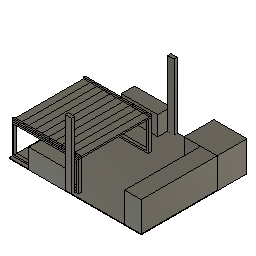
jumpy_camper_build (Autodesk Fusion 360 design; units mm, degrees)
part number: 2026-07-06-21-50-36-791
Autodesk Fusion 360 part; units mm, degrees
note: some values were not read from the file. Set by a fixed rule: which sketch regions a step uses.
sketch "Sketch1" plane through (0, 0, 0) normal (0, 0, 1) x (1, 0, 0)
  line L0 (0, 0) -> (2000, 0)
  line L1 (2000, 0) -> (2000, 1600)
  line L2 (2000, 1600) -> (0, 1600)
  line L3 (0, 1600) -> (0, 0)
  line L4 (2000, 800) -> (0, 800) construction
  line L5 (298.7393, 1600) -> (850, 1600)
  line L6 (850, 1600) -> (850, 1400)
  line L7 (850, 1400) -> (298.7393, 1400)
  line L8 (298.7393, 1400) -> (298.7393, 1600)
  line L9 (298.7393, 0) -> (850, 0)
  line L10 (850, 0) -> (850, 200)
  line L11 (850, 200) -> (298.7393, 200)
  line L12 (298.7393, 200) -> (298.7393, 0)
  line L13 (850, 1550) -> (946.8887, 1550)
  line L14 (946.8887, 1550) -> (946.8887, 1600)
  line L15 (946.8887, 1600) -> (850, 1600)
  line L16 (850, 1600) -> (850, 1550)
  line L17 (946.8887, 0) -> (850, 0)
  line L18 (850, 0) -> (850, 50)
  line L19 (850, 50) -> (946.8887, 50)
  line L20 (946.8887, 50) -> (946.8887, 0)
  dimension "d1" = 2000
  dimension "d2" = 1600
  dimension "d3" = 200
  dimension "d8" = 1500
  constraint horizontal L0
  constraint vertical L1
  constraint horizontal L2
  constraint vertical L3
  constraint coincident L0.start L3.end
  constraint midpoint L1 L4.start
  constraint midpoint L3 L4.end
  constraint horizontal L5
  constraint vertical L6
  constraint horizontal L7
  constraint vertical L8
  constraint coincident L2 L5.start
  constraint symmetric L4 L5.start L9.start
  constraint symmetric L4 L5.end L9.end
  constraint symmetric L4 L6.end L10.end
  constraint symmetric L4 L7.end L11.end
  constraint horizontal L13
  constraint vertical L14
  constraint horizontal L15
  constraint vertical L16
  constraint coincident L2 L14.end
  constraint coincident L6 L13.start
  constraint symmetric L4 L13.start L18.end
  constraint symmetric L4 L13.end L19.end
  constraint symmetric L4 L14.end L17.start
  measures "d1" distance of L0.start L0.end
  measures "d2" distance of L0.start L2.end
  measures "d3" distance of L5.end L6.end
  measures "d8" distance of L13 L19
extrude "Extrude1" add sketch "Sketch1" along normal blind 10 contours L0 L1 L2 L3 L6 L7 L8 L10 L11 L12 L13 L14 L19 L20 | L0 L10 L17 L18 L19 L20 | L2 L6 L13 L14 L15 L16 makes body 1
extrude "Extrude2" add sketch "Sketch1" along normal blind 300 contours L0 L9 L10 L11 L12 L18 | L2 L5 L6 L7 L8 L16 bodies 1
extrude "Extrude3" add sketch "Sketch1" along normal blind 1000 separate body contours L0 L10 L17 L18 L19 L20 | L2 L6 L13 L14 L15 L16 makes body 2 at (914.5925, 1550, 666.6667) makes body 3 at (914.5925, 50, 666.6667)
sketch "Sketch2" plane through (0, 0, 10) normal (0, 0, 1) x (-1, 0, 0)
  line L0 (-850, 0) -> (-2000, 0)
  line L1 (-2000, 0) -> (-2000, -1600)
  line L2 (-2000, -1600) -> (-850, -1600)
  line L3 (-850, -1600) -> (-850, -1400)
  line L4 (-850, -1400) -> (-298.7393, -1400)
  line L5 (-298.7393, -1400) -> (-298.7393, -1600)
  line L6 (-298.7393, -1600) -> (0, -1600)
  line L7 (0, -1600) -> (0, 0)
  line L8 (0, 0) -> (-298.7393, 0)
  line L9 (-298.7393, 0) -> (-298.7393, -200)
  line L10 (-298.7393, -200) -> (-850, -200)
  line L11 (-850, -200) -> (-850, 0)
  line L12 (0, -1400) -> (-1000, -1400)
  line L13 (-1000, -1400) -> (-1000, -1356)
  line L14 (-1000, -1356) -> (0, -1356)
  line L15 (0, -1356) -> (0, -1400)
  line L16 (-2000, -1600) -> (-1500, -1600)
  line L17 (-1500, -1600) -> (-1500, -1150)
  line L18 (-1500, -1150) -> (-2000, -1150)
  line L19 (-2000, -1150) -> (-2000, -1600)
  dimension "d11" = 44
  dimension "d14" = 500
  dimension "d15" = 450
  dimension "d18" = 1000
  constraint horizontal L12
  constraint vertical L13
  constraint horizontal L14
  constraint vertical L15
  constraint coincident L7 L12.start
  constraint horizontal L16
  constraint vertical L17
  constraint horizontal L18
  constraint vertical L19
  constraint coincident L1.end L2.start
  measures "d11" distance of L12.start L14.end
  measures "d14" distance of L1.end L16.end
  measures "d15" distance of L1.end L18.end
  measures "d18" distance of L13 L15
extrude "Extrude4" add sketch "Sketch2" along normal blind 24 separate body contours L4 L7 L12 L13 L14 L15 makes body 4
extrude "Extrude5" add sketch "Sketch2" along normal blind 450 contours L1 L2 L16 L17 L18 L19 bodies 1
sketch "Sketch3" plane through (0, 0, 34) normal (0, 0, 1) x (-1, 0, 0)
  line L0 (0, -1356) -> (-1000, -1356)
  line L1 (-1000, -1356) -> (-1000, -1400)
  line L2 (-1000, -1400) -> (0, -1400)
  line L3 (0, -1400) -> (0, -1356)
  line L4 (-1000, -1400) -> (-976, -1400)
  line L5 (-976, -1400) -> (-976, -1356)
  line L6 (-976, -1356) -> (-1000, -1356)
  line L7 (-1000, -1356) -> (-1000, -1400)
  dimension "d19" = 24
  constraint horizontal L4
  constraint vertical L5
  constraint horizontal L6
  constraint vertical L7
  constraint coincident L1.end L2.start
  measures "d19" distance of L1.end L4.end
extrude "Extrude6" add sketch "Sketch3" along normal blind 402 separate body contours L0 L1 L2 L4 L5 L6 L7 makes body 5
copy_body "CopyPasteBodies1" bodies 5 makes body 6
move_body "Move1" bodies 6 to x (1, 0, 0) y (0, 1, 0) z (0, 0, 1) at (-976, 0, 0)
copy_body "CopyPasteBodies2" bodies 4 makes body 7
move_body "Move2" bodies 7 to x (1, 0, 0) y (0, 1, 0) z (0, 0, 1) at (0, 0, 426)
combine "Combine1" operation add target body 4 tool bodies 5 6 7
ref_plane "WorkPlane1" through (1000, 800, 150) normal (0, -1, 0) x (1, 0, 0)
mirror "Mirror1" about plane through (1000, 800, 150) normal (0, -1, 0) of bodies 4 makes body 8
sketch "Sketch4" plane through (0, 0, 460) normal (0, 0, 1) x (-1, 0, 0)
  line L0 (0, -1356) -> (-1000, -1356)
  line L1 (-1000, -1356) -> (-1000, -1400)
  line L2 (-1000, -1400) -> (0, -1400)
  line L3 (0, -1400) -> (0, -1356)
  line L4 (0, -1400) -> (-1000, -1400)
  line L5 (-1000, -1400) -> (-1000, -1300)
  line L6 (-1000, -1300) -> (0, -1300)
  line L7 (0, -1300) -> (0, -1400)
  constraint horizontal L4
  constraint vertical L5
  constraint horizontal L6
  constraint vertical L7
  constraint coincident L2.end L3.start
extrude "Extrude7" add sketch "Sketch4" along normal blind 23 separate body makes body 9
copy_body "CopyPasteBodies3" bodies 9 makes body 10
copy_body "CopyPasteBodies4" bodies 10 makes body 11
move_body "Move3" bodies 11 to x (1, 0, 0) y (0, 1, 0) z (0, 0, 1) at (0, -100, 0)
copy_body "CopyPasteBodies5" bodies 10 11 makes body 12 makes body 13
move_body "Move4" bodies 12 13 to x (1, 0, 0) y (0, 1, 0) z (0, 0, 1) at (0, -200, 0)
copy_body "CopyPasteBodies6" bodies 10 11 makes body 14 makes body 15
move_body "Move5" bodies 14 15 to x (1, 0, 0) y (0, 1, 0) z (0, 0, 1) at (0, -400, 0)
copy_body "CopyPasteBodies7" bodies 10 11 makes body 16 makes body 17
move_body "Move6" bodies 16 17 to x (1, 0, 0) y (0, 1, 0) z (0, 0, 1) at (0, -600, 0)
copy_body "CopyPasteBodies8" bodies 10 11 makes body 18 makes body 19
move_body "Move7" bodies 18 19 to x (1, 0, 0) y (0, 1, 0) z (0, 0, 1) at (0, -800, 0)
copy_body "CopyPasteBodies9" bodies 10 11 makes body 20 makes body 21
move_body "Move8" bodies 20 21 to x (1, 0, 0) y (0, 1, 0) z (0, 0, 1) at (0, -1000, 0)
sketch "Sketch5" plane through (0, 0, 460) normal (0, 0, -1) x (1, 0, 0)
  line L0 (1000, -1300) -> (0, -1300)
  line L1 (0, -1300) -> (0, -1400)
  line L2 (0, -1400) -> (1000, -1400)
  line L3 (1000, -1400) -> (1000, -1300)
  line L4 (0, -1356) -> (44, -1356)
  line L5 (44, -1356) -> (44, -244)
  line L6 (44, -244) -> (0, -244)
  line L7 (0, -244) -> (0, -1356)
  point P0 (0, -1356)
  dimension "d26" = 44
  constraint horizontal L4
  constraint vertical L5
  constraint horizontal L6
  constraint vertical L7
  constraint coincident P0 L4.start
  measures "d26" distance of P0 L4.end
extrude "Extrude8" add sketch "Sketch5" along normal blind 24 separate body contours L0 L1 L4 L5 L7 | L0 L5 L6 L7 makes body 22
sketch "Sketch8" plane through (0, 0, 436) normal (0, 0, -1) x (1, 0, 0)
  line L0 (0, -244) -> (0, -1356)
  line L1 (0, -1356) -> (44, -1356)
  line L2 (44, -1356) -> (44, -244)
  line L3 (44, -244) -> (0, -244)
  circle A0 centre (15.3919, -268.552) radius 5
  circle A1 centre (11.7407, -456.5231) radius 5
  circle A2 centre (25, -675) radius 5
  circle A3 centre (25, -850) radius 5
  circle A4 centre (20.3714, -1058.8292) radius 5
  circle A5 centre (18.3231, -1241.9329) radius 5
  dimension "d29" = 10
  dimension "d30" = 10
  dimension "d31" = 10
  dimension "d32" = 10
  dimension "d33" = 10
  dimension "d34" = 10
  measures "d29" diameter of A0
  measures "d30" diameter of A1
  measures "d31" diameter of A2
  measures "d32" diameter of A3
  measures "d33" diameter of A4
  measures "d34" diameter of A5
extrude "Extrude9" cut sketch "Sketch8" against normal blind 90 contours A0 | A1 | A2 | A3 | A4 | A5 bodies 11 13 15 17 19 21 22
move_body "Move9" bodies 8 4 to x (1, 0, 0) y (0, 1, 0) z (0, 0, 1) at (0, -150, 0)
move_body "Move10" bodies 9 22 12 20 19 11 14 10 17 16 13 15 21 18 to x (1, 0, 0) y (0, 1, 0) z (0, 0, 1) at (0, -150, 0)
delete_body "RemoveBody1" bodies 10
delete_body "RemoveBody2" bodies 9
move_body "Move11" bodies 4 to x (1, 0, 0) y (0, 1, 0) z (0, 0, 1) at (0, -100, 0)
extrude "Extrude10" cut 1 faces at (14.6667, 1206, 452) along direction (0, -1, 0) blind 100 on bodies 22 bodies 4 22
delete_body "RemoveBody3" bodies 11
delete_body "RemoveBody4" bodies 12
delete_body "RemoveBody5" bodies 13
delete_body "RemoveBody6" bodies 14
delete_body "RemoveBody7" bodies 15
delete_body "RemoveBody8" bodies 16
delete_body "RemoveBody9" bodies 17
delete_body "RemoveBody10" bodies 18
delete_body "RemoveBody11" bodies 19
delete_body "RemoveBody12" bodies 20
delete_body "RemoveBody13" bodies 21
delete_body "RemoveBody14" bodies 22
extrude "Extrude11" add 1 faces at (44, 1135.3333, 452) along direction (-1, 0, 0) blind 44 on bodies 4 bodies 4
sketch "Sketch9" plane through (0, 0, 460) normal (0, 0, 1) x (-1, 0, 0)
  line L0 (0, -1106) -> (-1000, -1106)
  line L1 (-1000, -1106) -> (-1000, -1150)
  line L2 (-1000, -1150) -> (0, -1150)
  line L3 (0, -1150) -> (0, -1106)
  line L4 (0, -1150) -> (-100, -1150)
  line L5 (-100, -1150) -> (-100, -50)
  line L6 (-100, -50) -> (0, -50)
  line L7 (0, -50) -> (0, -1150)
  dimension "d41" = 100
  constraint horizontal L4
  constraint vertical L5
  constraint horizontal L6
  constraint vertical L7
  constraint coincident L2.end L3.start
  measures "d41" distance of L2.end L4.end
extrude "Extrude12" add sketch "Sketch9" along normal blind 23 separate body contours L0 L2 L3 L4 L5 L7 | L0 L5 L6 L7 makes body 23
copy_body "CopyPasteBodies10" bodies 23 makes body 24
move_body "Move12" bodies 24 to x (1, 0, 0) y (0, 1, 0) z (0, 0, 1) at (100, 0, 0)
copy_body "CopyPasteBodies11" bodies 23 24 makes body 25 makes body 26
move_body "Move13" bodies 25 26 to x (1, 0, 0) y (0, 1, 0) z (0, 0, 1) at (200, 0, 0)
copy_body "CopyPasteBodies12" bodies 23 24 25 26 makes body 27 makes body 28 makes body 29 makes body 30
move_body "Move14" bodies 27 28 29 30 to x (1, 0, 0) y (0, 1, 0) z (0, 0, 1) at (400, 0, 0)
copy_body "CopyPasteBodies13" bodies 28 29 30 makes body 31 makes body 32 makes body 33
move_body "Move15" bodies 31 32 33 to x (1, 0, 0) y (0, 1, 0) z (0, 0, 1) at (300, 0, 0)
delete_body "RemoveBody15" bodies 33
sketch "Sketch10" plane through (0, 0, 483) normal (0, 0, 1) x (-1, 0, 0)
  line L0 (0, -50) -> (-100, -50)
  line L1 (-100, -50) -> (-100, -1150)
  line L2 (-100, -1150) -> (0, -1150)
  line L3 (0, -1150) -> (0, -50)
  line L4 (0, -50) -> (-1000, -50)
  line L5 (-1000, -50) -> (-1000, -74)
  line L6 (-1000, -74) -> (0, -74)
  line L7 (0, -74) -> (0, -50)
  dimension "d44" = 24
  constraint horizontal L4
  constraint vertical L5
  constraint horizontal L6
  constraint vertical L7
  constraint coincident L0.start L3.end
  measures "d44" distance of L0.start L6.end
extrude "Extrude13" add sketch "Sketch10" along normal blind 24 separate body contours L0 L1 L3 L4 L6 L7 | L1 L4 L5 L6 makes body 34
sketch "Sketch11" plane through (0, 0, 507) normal (0, 0, 1) x (-1, 0, 0)
  line L0 (0, -74) -> (0, -50)
  line L1 (0, -50) -> (-1000, -50)
  line L2 (-1000, -50) -> (-1000, -74)
  line L3 (-1000, -74) -> (0, -74)
  circle A0 centre (-150, -60) radius 5
  circle A1 centre (-350, -60) radius 5
  circle A2 centre (-550, -60) radius 5
  circle A3 centre (-740, -60) radius 5
  circle A4 centre (-950, -60) radius 5
  dimension "d47" = 10
  dimension "d48" = 10
  dimension "d49" = 10
  dimension "d50" = 10
  dimension "d51" = 10
  measures "d47" diameter of A0
  measures "d48" diameter of A1
  measures "d49" diameter of A2
  measures "d50" diameter of A3
  measures "d51" diameter of A4
extrude "Extrude14" cut sketch "Sketch11" against normal blind 70 contours A0 | A1 | A2 | A3 | A4 bodies 8 24 26 28 30 32 34
copy_body "CopyPasteBodies14" bodies 34 makes body 35
move_body "Move16" bodies 35 to x (1, 0, 0) y (0, 1, 0) z (0, 0, 1) at (0, 1076, 0)
sketch "Sketch12" plane through (0, 0, 10) normal (0, 0, 1) x (-1, 0, 0)
  line L0 (-1500, -1150) -> (-1500, -1600)
  line L1 (-1500, -1600) -> (-850, -1600)
  line L2 (-850, -1600) -> (-850, -1400)
  line L3 (-850, -1400) -> (-298.7393, -1400)
  line L4 (-298.7393, -1400) -> (-298.7393, -1600)
  line L5 (-298.7393, -1600) -> (0, -1600)
  line L6 (0, -1600) -> (0, 0)
  line L7 (0, 0) -> (-298.7393, 0)
  line L8 (-298.7393, 0) -> (-298.7393, -200)
  line L9 (-298.7393, -200) -> (-850, -200)
  line L10 (-850, -200) -> (-850, 0)
  line L11 (-850, 0) -> (-2000, 0)
  line L12 (-2000, 0) -> (-2000, -1150)
  line L13 (-2000, -1150) -> (-1500, -1150)
  line L14 (-2000, -1150) -> (-1750, -1150)
  line L15 (-1750, -1150) -> (-1750, 0)
  line L16 (-1750, 0) -> (-2000, 0)
  line L17 (-2000, 0) -> (-2000, -1150)
  dimension "d54" = 250
  constraint horizontal L14
  constraint vertical L15
  constraint horizontal L16
  constraint vertical L17
  constraint coincident L12.end L13.start
  measures "d54" distance of L12.end L14.end
extrude "Extrude15" add sketch "Sketch12" along normal blind 450 separate body contours L11 L12 L13 L14 L15 L16 L17 makes body 36
equation "d20 = 450 mm - 48 mm"
